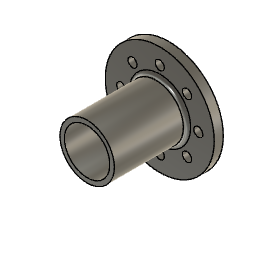
Flange (Autodesk Fusion 360 design; units mm, degrees)
Autodesk Fusion 360 part; units mm, degrees
sketch "Sketch1" plane through (0, 0, 0) normal (0, 1, 0) x (1, 0, 0)
  circle A0 centre (0, 0) radius 38.1
  dimension "d1" = 76.2
  constraint coincident A0.centre origin
  measures "d1" diameter of A0
extrude "Extrude1" add sketch "Sketch1" against normal blind 6.35
sketch "Sketch2" plane through (0, -6.35, 0) normal (0, -1, 0) x (1, 0, 0)
  circle A0 centre (0, 0) radius 38.1
  circle A1 centre (0, 0) radius 15.875
  dimension "d4" = 31.75
  constraint concentric A0 A1
  measures "d4" diameter of A1
extrude "Extrude2" cut sketch "Sketch2" against normal blind 83.82 contours A1
sketch "Sketch3" plane through (0, -6.35, 0) normal (0, -1, 0) x (1, 0, 0)
  circle A0 centre (0, 0) radius 15.875
  circle A1 centre (0, 0) radius 38.1
  circle A2 centre (0, 0) radius 15.875
  circle A3 centre (0, 0) radius 19.05
  dimension "d7" = 31.75
  dimension "d8" = 38.1
  constraint concentric A0 A2
  constraint concentric A2 A3
  measures "d7" diameter of A2
  measures "d8" diameter of A3
extrude "Extrude3" add sketch "Sketch3" along normal blind 50.8 contours A3
fillet "Fillet1" radius 2.54 1 edges at (-17.7608, -6.35, 6.8888)
sketch "Sketch4" plane through (0, 0, 0) normal (0, 1, 0) x (-1, 0, 0)
  circle A0 centre (0, 0) radius 15.875
  circle A1 centre (0, 0) radius 38.1
  circle A2 centre (0, 26.9875) radius 3.175
  circle A3 centre (-19.083, 19.083) radius 3.175
  circle A4 centre (-26.9875, 0) radius 3.175
  circle A5 centre (-19.083, -19.083) radius 3.175
  circle A6 centre (0, -26.9875) radius 3.175
  circle A7 centre (19.083, -19.083) radius 3.175
  circle A8 centre (26.9875, 0) radius 3.175
  circle A9 centre (19.083, 19.083) radius 3.175
  dimension "d13" = 6.35
  dimension "d15" = 360
  measures "d13" diameter of A2
extrude "Extrude4" cut sketch "Sketch4" against normal blind 76.2 contours A2 | A3 | A4 | A5 | A6 | A7 | A8 | A9
sketch "Sketch5" plane through (0, 0, 0) normal (0, 1, 0) x (-1, 0, 0)
  circle A0 centre (0, 26.9875) radius 3.175
  circle A1 centre (0, -26.9875) radius 3.175
  circle A2 centre (19.083, -19.083) radius 3.175
  circle A3 centre (-19.083, 19.083) radius 3.175
  circle A4 centre (19.083, 19.083) radius 3.175
  circle A5 centre (-19.083, -19.083) radius 3.175
  circle A6 centre (26.9875, 0) radius 3.175
  circle A7 centre (-26.9875, 0) radius 3.175
  circle A8 centre (0, 0) radius 15.875
  circle A9 centre (0, 0) radius 38.1
  line L0 (-2.54, 15.875) -> (-2.54, -15.875)
  line L1 (2.54, 15.875) -> (2.54, -15.875)
  arc A10 (-2.54, -15.6705) -> (2.54, -15.6705) centre (0, 0) ccw
  arc A11 (2.54, 15.6705) -> (-2.54, 15.6705) centre (0, 0) ccw
  constraint concentric A8 A10
  constraint coincident L0 A11.end
  constraint coincident L0 A10.start
  constraint coincident L1 A10.end
  constraint coincident L1 A11.start
  constraint concentric A10 A11
extrude "Extrude5" add sketch "Sketch5" against normal blind 12.7 contours A8 L0 L1 A10 A11
